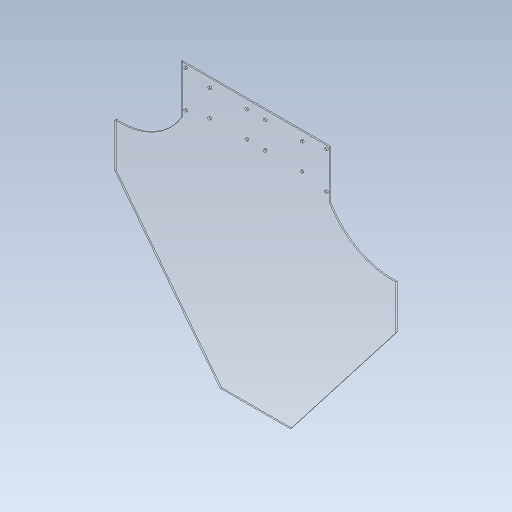
# Autodesk Inventor part: シールド
Saved by Autodesk Inventor 2020 (Build 240168000, 168)
## iProperties
Created: 2020-02-13
Part Number: シールド
Material: ポリカーボネート、クリア
Document SubType Name: Modeling
Designer: tanjihayato
Density: 1.2 g/cm^3
Appearance: ポリカーボネート - クリア
Mass: 116.24 g
Surface Area: 1308.71 cm^2
Volume: 96.8663 cm^3
Author: tanjihayato
Autodesk Inventor part; units mm, degrees
ref_plane "YZ Plane" through (0, 0, 0) normal (1, 0, 0) x (0, 1, 0)
ref_plane "XZ Plane" through (0, 0, 0) normal (0, 1, 0) x (-1, 0, 0)
ref_plane "XY Plane" through (0, 0, 0) normal (0, 0, 1) x (1, 0, 0)
sketch "スケッチ1" plane through (0, 0, 0) normal (0, 0, 1) x (1, 0, 0)
  line L0 (0, 0) -> (3, 0)
  line L1 (3, 0) -> (3, -15)
  line L2 (3, -15) -> (0, -15)
  line L3 (0, -15) -> (0, 0)
  line L4 (-9, 0) -> (-6, 0)
  line L5 (-6, 0) -> (-6, -15)
  line L6 (-6, -15) -> (-9, -15)
  line L7 (-9, -15) -> (-9, 0)
  line L8 (0, -30) -> (3, -30)
  line L9 (3, -30) -> (3, -45)
  line L10 (3, -45) -> (0, -45)
  line L11 (0, -45) -> (0, -30)
  line L12 (-9, -30) -> (-6, -30)
  line L13 (-6, -30) -> (-6, -45)
  line L14 (-6, -45) -> (-9, -45)
  line L15 (-9, -45) -> (-9, -30)
  line L16 (-87.5, 3) -> (81.5, 3)
  line L17 (-87.5, 3) -> (-87.5, -48)
  line L18 (-87.5, -48) -> (81.5, -48)
  line L19 (81.5, -48) -> (81.5, 3)
  circle A0 centre (-83, -1.5) radius 1.5
  circle A1 centre (77, -1.5) radius 1.5
  circle A2 centre (77, -43.5) radius 1.5
  circle A3 centre (-83, -43.5) radius 1.5
  circle A4 centre (3, -1.05) radius 1.05
  circle A5 centre (3, -13.95) radius 1.05
  circle A6 centre (0, -13.95) radius 1.05
  circle A7 centre (0, -1.05) radius 1.05
  circle A8 centre (-6, -1.05) radius 1.05
  circle A9 centre (-6, -13.95) radius 1.05
  circle A10 centre (-9, -13.95) radius 1.05
  circle A11 centre (-9, -1.05) radius 1.05
  circle A12 centre (-6, -31.05) radius 1.05
  circle A13 centre (-6, -43.95) radius 1.05
  circle A14 centre (-9, -43.95) radius 1.05
  circle A15 centre (-9, -31.05) radius 1.05
  circle A16 centre (0, -31.05) radius 1.05
  circle A17 centre (3, -31.05) radius 1.05
  circle A18 centre (3, -43.95) radius 1.05
  circle A19 centre (0, -43.95) radius 1.05
  circle A20 centre (-13.5, -7.5) radius 1.5
  circle A21 centre (7.5, -7.5) radius 1.5
  circle A22 centre (7.5, -37.5) radius 1.5
  circle A23 centre (-13.5, -37.5) radius 1.5
  line L20 (45, -30) -> (45, -45)
  line L21 (45, -45) -> (42, -45)
  circle A24 centre (42, -43.95) radius 1.05
  line L22 (42, -45) -> (42, -30)
  circle A25 centre (45, -43.95) radius 1.05
  line L23 (42, 0) -> (45, 0)
  line L24 (45, 0) -> (45, -15)
  line L25 (45, -15) -> (42, -15)
  line L26 (42, -15) -> (42, 0)
  circle A26 centre (45, -1.05) radius 1.05
  circle A27 centre (42, -1.05) radius 1.05
  circle A28 centre (42, -13.95) radius 1.05
  circle A29 centre (45, -13.95) radius 1.05
  line L27 (42, -30) -> (45, -30)
  circle A30 centre (45, -31.05) radius 1.05
  circle A31 centre (42, -31.05) radius 1.05
  circle A32 centre (49.5, -37.5) radius 1.5
  circle A33 centre (49.5, -7.5) radius 1.5
  line L28 (-51, -15) -> (-51, 0)
  line L29 (-48, -30) -> (-48, -45)
  line L30 (-51, -45) -> (-51, -30)
  line L31 (-48, 0) -> (-48, -15)
  circle A34 centre (-48, -31.05) radius 1.05
  circle A35 centre (-48, -43.95) radius 1.05
  circle A36 centre (-51, -13.95) radius 1.05
  circle A37 centre (-55.5, -7.5) radius 1.5
  circle A38 centre (-48, -1.05) radius 1.05
  circle A39 centre (-51, -1.05) radius 1.05
  circle A40 centre (-48, -13.95) radius 1.05
  line L32 (-48, -45) -> (-51, -45)
  line L33 (-51, -30) -> (-48, -30)
  line L34 (-51, 0) -> (-48, 0)
  line L35 (-48, -15) -> (-51, -15)
  circle A41 centre (-51, -43.95) radius 1.05
  circle A42 centre (-51, -31.05) radius 1.05
  circle A43 centre (-55.5, -37.5) radius 1.5
  point P0 (0, -42.9)
  point P1 (0, -32.1)
  point P2 (3, -32.1)
  point P3 (3, -42.9)
  point P4 (0, -2.1)
  point P5 (3, -2.1)
  point P6 (3, -12.9)
  point P7 (0, -12.9)
  point P8 (-9, -2.1)
  point P9 (-6, 0)
  point P10 (-6, -2.1)
  point P11 (-6, -12.9)
  point P12 (-9, -12.9)
  point P13 (-9, -32.1)
  point P14 (-6, -32.1)
  point P15 (-6, -42.9)
  point P16 (-9, -42.9)
  point P17 (-4.9275, 0)
  point P18 (1, -30)
  point P19 (-51, -32.1)
  point P20 (-48, -32.1)
  point P21 (-48, -42.9)
  point P22 (-51, -42.9)
  point P23 (42, -12.9)
  point P24 (42, -2.1)
  point P25 (45, -2.1)
  point P26 (45, -12.9)
  point P27 (42, -32.1)
  point P28 (45, -32.1)
  point P29 (45, -42.9)
  point P30 (42, -42.9)
  point P31 (-51, -12.9)
  point P32 (-51, -2.1)
  point P33 (-51, 0)
  point P34 (-48, -2.1)
  point P35 (-48, -12.9)
  dimension "d0" = 3
  dimension "d1" = 15
  dimension "d2" = 3
  dimension "d3" = 15
  dimension "d4" = 3
  dimension "d5" = 15
  dimension "d6" = 3
  dimension "d7" = 15
  dimension "d8" = 15
  dimension "d9" = 6
  dimension "d10" = 3
  dimension "d11" = 3
  dimension "d12" = 3
  dimension "d13" = 3
  dimension "d14" = 3
  dimension "d15" = 3
  dimension "d16" = 4.5
  dimension "d17" = 4.5
  dimension "d18" = 4.5
  dimension "d19" = 4.5
  dimension "d20" = 4.5
  dimension "d21" = 4.5
  dimension "d22" = 4.5
  dimension "d23" = 4.5
  dimension "d24" = 160
  dimension "d25" = 74
  dimension "d26" = 2.1
  dimension "d27" = 3
  dimension "d28" = 3
  dimension "d29" = 3
  dimension "d30" = 3
  dimension "d31" = 4.5
  dimension "d32" = 4.5
  dimension "d33" = 4.5
  dimension "d34" = 4.5
  dimension "d35" = 7.5
  dimension "d36" = 7.5
  dimension "d37" = 7.5
  dimension "d38" = 7.5
  dimension "d39" = 3
  dimension "d40" = 15
  dimension "d41" = 3
  dimension "d42" = 15
  dimension "d43" = 15
  dimension "d44" = 2.1
  dimension "d45" = 3
  dimension "d46" = 3
  dimension "d47" = 4.5
  dimension "d48" = 4.5
  dimension "d49" = 7.5
  dimension "d50" = 7.5
  dimension "d51" = 3
  dimension "d52" = 15
  dimension "d53" = 3
  dimension "d54" = 15
  dimension "d55" = 3
  dimension "d56" = 3
  dimension "d57" = 4.5
  dimension "d58" = 4.5
  dimension "d59" = 7.5
  dimension "d60" = 7.5
  dimension "d61" = 3
  dimension "d62" = 90
  dimension "d63" = 36.5
  constraints: 72 end point, 44 centre point, 40 point on line, 32 tangent, 29 equal radius, 16 parallel, 10 perpendicular, 9 horizontal, 2 collinear, 1 vertical
  measures "d0" distance of L1.end L2.end
  measures "d1" distance of L0.end L1.end
  measures "d2" distance of L5.end L6.end
  measures "d3" distance of L4.end L5.end
  measures "d4" distance of L9.end L10.end
  measures "d5" distance of L8.end L9.end
  measures "d6" distance of L13.end L14.end
  measures "d7" distance of L12.end L13.end
  measures "d8" distance between parallel lines of L8 L2
  measures "d9" distance between parallel lines of L13 L11
  measures "d10" distance between parallel lines of L4 L16
  measures "d11" distance between parallel lines of L18 L10
  measures "d12" diameter of A0
  measures "d13" diameter of A1
  measures "d14" diameter of A2
  measures "d15" diameter of A3
  measures "d16" distance from line of A0.centre L16
  measures "d17" distance from line of L17 A0.centre
  measures "d18" distance from line of L18 A3.centre
  measures "d19" distance from line of L17 A3.centre
  measures "d20" distance from line of L18 A2.centre
  measures "d21" distance from line of L19 A2.centre
  measures "d22" distance from line of L19 A1.centre
  measures "d23" distance from line of L16 A1.centre
  measures "d24" distance of A1.centre A0.centre
  measures "d25" distance from line of L1 A1.centre
  measures "d26" diameter of A4
  measures "d27" diameter of A20
  measures "d28" diameter of A21
  measures "d29" diameter of A22
  measures "d30" diameter of A23
  measures "d31" distance from line of A20.centre L7
  measures "d32" distance from line of L1 A21.centre
  measures "d33" distance from line of L9 A22.centre
  measures "d34" distance from line of L15 A23.centre
  measures "d35" distance from line of A21.centre L0
  measures "d36" distance from line of A20.centre L4
  measures "d37" distance from line of L14 A23.centre
  measures "d38" distance from line of L10 A22.centre
  measures "d39" distance of L24.end L25.end
  measures "d40" distance of L23.end L24.end
  measures "d41" distance of L20.end L21.end
  measures "d42" distance of L20.start L20.end
  measures "d43" distance between parallel lines of L27 L25
  measures "d44" diameter of A26
  measures "d45" diameter of A33
  measures "d46" diameter of A32
  measures "d47" distance from line of L24 A33.centre
  measures "d48" distance from line of L20 A32.centre
  measures "d49" distance from line of A33.centre L23
  measures "d50" distance from line of L21 A32.centre
  measures "d51" distance of L31.end L28.start
  measures "d52" distance of L31.start L31.end
  measures "d53" distance of L29.end L30.start
  measures "d54" distance of L29.start L29.end
  measures "d55" diameter of A37
  measures "d56" diameter of A43
  measures "d57" distance from line of A37.centre L28
  measures "d58" distance from line of L30 A43.centre
  measures "d59" distance from line of A37.centre L34
  measures "d60" distance from line of L32 A43.centre
  measures "d61" distance between parallel lines of L18 L21
  measures "d62" distance between parallel lines of L26 L31
  measures "d63" distance between parallel lines of L19 L24
sketch "スケッチ2" plane through (0, 0, 0) normal (0, 0, 1) x (1, 0, 0)
  circle A0 centre (-83, -1.5) radius 1.5 projected
  circle A1 centre (-83, -43.5) radius 1.5 projected
  circle A2 centre (-55.5, -7.5) radius 1.5 projected
  circle A3 centre (-55.5, -37.5) radius 1.5 projected
  circle A4 centre (-13.5, -37.5) radius 1.5 projected
  circle A5 centre (-13.5, -7.5) radius 1.5 projected
  circle A6 centre (7.5, -7.5) radius 1.5 projected
  circle A7 centre (7.5, -37.5) radius 1.5 projected
  circle A8 centre (49.5, -37.5) radius 1.5 projected
  circle A9 centre (49.5, -7.5) radius 1.5 projected
  circle A10 centre (77, -1.5) radius 1.5 projected
  circle A11 centre (77, -43.5) radius 1.5 projected
  line L0 (-87.5, 3) -> (81.5, 3) projected
  line L1 (-87.5, 3) -> (-87.5, -52.3382)
  line L2 (81.5, 3) -> (81.5, -52.3382)
  line L3 (-43, -297) -> (37, -297)
  line L4 (-43, -297) -> (-163, -142.321)
  line L5 (37, -297) -> (157, -142.321)
  line L6 (157, -142.321) -> (157, -92.4008)
  line L7 (-163, -142.321) -> (-163, -92.4008)
  arc A12 (-163, -92.4008) -> (-87.5, -52.3382) centre (-157.9321, -10.7785) ccw
  arc A13 (81.5, -52.3382) -> (157, -92.4008) centre (151.9321, -10.7785) ccw
  point P0 (0, 0)
  dimension "d66" = 80
  dimension "d67" = 300
  dimension "d68" = 44.5
  dimension "d69" = 44.5
  dimension "d70" = 320
  dimension "d71" = 75.5
  dimension "d72" = 75.5
  constraints: 14 end point, 4 point on circle, 4 vertical, 3 equal length, 2 centre point, 1 equal radius, 1 horizontal
  measures "d66" distance of L3.start L3.end
  measures "d67" distance between parallel lines of L3 L0
  measures "d68" distance from line of L3.end L2
  measures "d69" distance from line of L3.start L1
  measures "d70" distance between parallel lines of L7 L6
  measures "d71" distance between parallel lines of L6 L2
  measures "d72" distance between parallel lines of L7 L1
extrude "押し出し1" add sketch "スケッチ2" along normal blind 1.5
sketch "スケッチ3" plane through (0, 0, 1.5) normal (0, 0, 1) x (1, 0, 0)
  arc A0 (81.5, -62.77) -> (157, -104.1946) centre (152.6935, -22.5286) ccw projected
  line L0 (81.5, -62.77) -> (81.5, 3) projected
  line L1 (81.5, 3) -> (-87.5, 3) projected
  line L2 (-87.5, 3) -> (-87.5, -62.77) projected
  arc A1 (-163, -104.1946) -> (-87.5, -62.77) centre (-158.6935, -22.5286) ccw projected
  line L3 (-163, -104.1946) -> (-163, -142.321) projected
  line L4 (-163, -142.321) -> (-43, -297) projected
  line L5 (-43, -297) -> (37, -297) projected
  line L6 (37, -297) -> (157, -142.321) projected
  line L7 (157, -142.321) -> (157, -104.1946) projected
  circle A2 centre (77, -43.5) radius 1.5 projected
  circle A3 centre (49.5, -7.5) radius 1.5 projected
  circle A4 centre (7.5, -37.5) radius 1.5 projected
  circle A5 centre (7.5, -7.5) radius 1.5 projected
  circle A6 centre (-13.5, -7.5) radius 1.5 projected
  circle A7 centre (-13.5, -37.5) radius 1.5 projected
  circle A8 centre (-55.5, -37.5) radius 1.5 projected
  circle A9 centre (-55.5, -7.5) radius 1.5 projected
  circle A10 centre (-83, -43.5) radius 1.5 projected
  circle A11 centre (-83, -1.5) radius 1.5 projected
  circle A12 centre (49.5, -37.5) radius 1.5 projected
  circle A13 centre (77, -1.5) radius 1.5 projected
  line L8 (81.5, 3) -> (-87.5, 3) projected
  line L9 (-87.5, 3) -> (-57.4301, 94.7393)
  line L10 (-57.4301, 94.7393) -> (-30.5041, 94.7393)
  line L11 (-30.5041, 94.7393) -> (-30.5041, 42.9458)
  line L12 (-30.5041, 42.9458) -> (24.5041, 42.9458)
  line L13 (24.5041, 42.9458) -> (24.5041, 94.7393)
  line L14 (24.5041, 94.7393) -> (51.4301, 94.7393)
  line L15 (51.4301, 94.7393) -> (81.5, 3)
  point P0 (0, 0)
  dimension "d75" = 56.9959
  dimension "d76" = 56.9959
  constraints: 14 end point, 4 perpendicular, 1 collinear, 1 equal length, 1 parallel
  measures "d75" distance from line of L13 L0.end
  measures "d76" distance from line of L1.end L11
equation "\"d69\" = d68"
equation "\"d72\" = d71"
equation "\"d76\" = d75"
